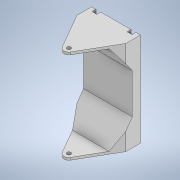
# Autodesk Inventor part: Y_axis
Saved by Autodesk Inventor 2020 (Build 240168000, 168)
## iProperties
Created: 2020-05-02
Part Number: Y_axis
Material: Generic
Document SubType Name: Modeling
Designer: zhang
Density: 1 g/cm^3
Appearance: Default
Author: zhang
Autodesk Inventor part; units mm, degrees
ref_plane "YZ Plane" through (0, 0, 0) normal (1, 0, 0) x (0, 1, 0)
ref_plane "XZ Plane" through (0, 0, 0) normal (0, 1, 0) x (-1, 0, 0)
ref_plane "XY Plane" through (0, 0, 0) normal (0, 0, 1) x (1, 0, 0)
sketch "Sketch1" plane through (0, 0, 0) normal (0, 1, 0) x (-1, 0, 0)
  line L0 (0, 26.7471) -> (0, -19.6773)
  circle A0 centre (0, 0) radius 8
  line L1 (17.3205, 10) -> (100, -133.2051)
  line L2 (100, -133.2051) -> (0, -133.2051) construction
  line L3 (43.971, 0) -> (-53.4185, 0)
  line L4 (-17.3205, 10) -> (-100, -133.2051)
  line L5 (-100, -133.2051) -> (0, -133.2051) construction
  line L6 (-43.971, 0) -> (53.4185, 0)
  line L7 (100, -133.2051) -> (100, -193.2051)
  line L8 (100, -193.2051) -> (-100, -193.2051)
  line L9 (-100, -193.2051) -> (-100, -133.2051)
  arc A1 (17.3205, 10) -> (-17.3205, 10) centre (0, 0) ccw
  point P0 (0, 40)
  dimension "d0" = 16
  dimension "d2" = 100
  dimension "d3" = 80
  dimension "d4" = 60
  dimension "d5" = 60
  dimension "d6" = 20
  constraints: 20 end point, 4 point on line, 3 perpendicular, 3 symmetric about line, 3 vertical, 2 centre point, 2 horizontal, 2 point on circle, 2 tangent, 1 coincident
  measures "d0" diameter of A0
  measures "d2" distance of L1.end L2.end
  measures "d3" diameter of point (0, 40) L3
  measures "d4" angle of L2 L1
  measures "d5" distance of L8.end L4.end
  measures "d6" radius of A1
extrude "Extrusion1" add sketch "Sketch1" along normal mid plane 384 contours A1 L1 L3 A0 L0 | L0 A0 L3 L4 A1 | L3 L1 L7 L8 L9 L4 A0
sketch "Sketch2" plane through (0, 0, 0) normal (1, 0, 0) x (0, 1, 0)
  line L0 (0, 110.6795) -> (0, -260.886)
  line L1 (-192, 20) -> (192, 20) projected
  line L2 (-182, 20) -> (-182, -90)
  line L3 (-182, -90) -> (-82.0296, -160)
  line L4 (-82.0296, -160) -> (0, -160)
  line L5 (-182, 20) -> (0, 20)
  line L6 (-192, 10) -> (-192, -133.2051) projected
  line L7 (182, 20) -> (182, -90)
  line L8 (182, -90) -> (82.0296, -160)
  line L9 (82.0296, -160) -> (0, -160)
  line L10 (182, 20) -> (0, 20)
  point P0 (0, 0)
  dimension "d9" = 10
  dimension "d10" = 180
  dimension "d11" = 110
  dimension "d12" = 145
  constraints: 16 end point, 3 horizontal alignment, 1 horizontal, 1 midpoint, 1 point on line, 1 vertical, 4 other
  measures "d9" distance between parallel lines of L6 L2
  measures "d10" distance between parallel lines of L4 L1
  measures "d11" distance of L2.start L2.end
  measures "d12" angle of L4 L3
extrude "Extrusion2" cut sketch "Sketch2" along normal through all both and the other way through all
sketch "Sketch3" plane through (0, 192, 0) normal (0, 1, 0) x (1, 0, 0)
  circle A0 centre (0, 0) radius 8 projected
  line L0 (0, 0) -> (0, 264.7733)
  line L1 (-100, 193.2051) -> (100, 193.2051) projected
  line L2 (-82, 193.2051) -> (-62, 193.2051)
  line L3 (-62, 193.2051) -> (-62, 177.2051)
  line L4 (-62, 177.2051) -> (-82, 177.2051)
  line L5 (-82, 177.2051) -> (-82, 193.2051)
  line L6 (-100, 193.2051) -> (-100, 133.2051) projected
  line L7 (82, 193.2051) -> (62, 193.2051)
  line L8 (62, 193.2051) -> (62, 177.2051)
  line L9 (62, 177.2051) -> (82, 177.2051)
  line L10 (82, 177.2051) -> (82, 193.2051)
  dimension "d15" = 18
  dimension "d16" = 20
  dimension "d17" = 16
  constraints: 18 end point, 4 symmetric about line, 2 parallel, 1 horizontal, 1 perpendicular, 1 point on line, 1 vertical
  measures "d15" distance between parallel lines of L6 L5
  measures "d16" distance of L3.end L4.end
  measures "d17" distance of L2.end L3.end
extrude "Extrusion3" cut sketch "Sketch3" against normal through all contours L3 L4 L5 L1 | L1 L10 L9 L8
body "Solid1"
